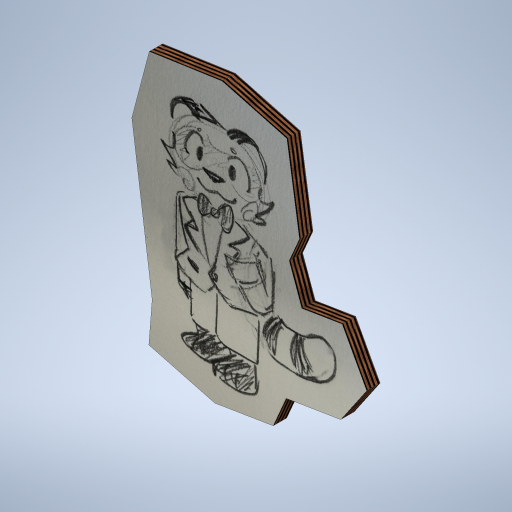
# Autodesk Inventor part: petti
Saved by Autodesk Inventor 2023 (Build 270158000, 158)
## iProperties
Created: 2024-07-02
Part Number: petti
Material: Generic
Document SubType Name: Modeling
Designer: Student-27
Density: 1 g/cm^3
Appearance: Default
Author: Student-27
Autodesk Inventor part; units mm, degrees
ref_plane "YZ Plane" through (0, 0, 0) normal (1, 0, 0) x (0, 1, 0)
ref_plane "XZ Plane" through (0, 0, 0) normal (0, 1, 0) x (-1, 0, 0)
ref_plane "XY Plane" through (0, 0, 0) normal (0, 0, 1) x (1, 0, 0)
sketch "Sketch1" plane through (0, 0, 0) normal (0, 0, 1) x (1, 0, 0)
  line L0 (-7.5953, 9.4076) -> (792.5047, 9.4076) construction
  line L1 (792.5047, 9.4076) -> (792.5047, -1057.3924) construction
  line L2 (792.5047, -1057.3924) -> (-7.5953, -1057.3924) construction
  line L3 (-7.5953, -1057.3924) -> (-7.5953, 9.4076) construction
  line L4 (391.2026, -306.0369) -> (514.2891, -338.9885)
  line L5 (514.2891, -338.9885) -> (538.0727, -491.3852)
  line L6 (538.0727, -491.3852) -> (518.6531, -536.4419)
  line L7 (518.6531, -536.4419) -> (542.5289, -602.5594)
  line L8 (542.5289, -602.5594) -> (618.6657, -590.1287)
  line L9 (618.6657, -590.1287) -> (664.9302, -676.146)
  line L10 (664.9302, -676.146) -> (615.9468, -747.6618)
  line L11 (615.9468, -747.6618) -> (513.1068, -764.4524)
  line L12 (513.1068, -764.4524) -> (488.4994, -821.5458)
  line L13 (488.4994, -821.5458) -> (378.1142, -839.5683)
  line L14 (378.1142, -839.5683) -> (253.8056, -806.7882)
  line L15 (253.8056, -806.7882) -> (260.0674, -729.2793)
  line L16 (260.0674, -729.2793) -> (221.6415, -451.1978)
  line L17 (221.6415, -451.1978) -> (254.5109, -326.5507)
  line L18 (254.5109, -326.5507) -> (391.9348, -306.2329)
  line L19 (221.6415, -306.2329) -> (664.9302, -306.2329)
  line L20 (664.9302, -306.2329) -> (664.9302, -840.0021)
  line L21 (664.9302, -840.0021) -> (221.6415, -840.0021)
  line L22 (221.6415, -840.0021) -> (221.6415, -306.2329)
  point P0 (0, 0)
  dimension "d15" = 533.7692
  dimension "d18" = 443.2887
  constraints: 38 end point, 5 parallel, 2 perpendicular, 2 point on line, 1 horizontal, 2 other
  measures "d15" distance of L21.end L19.start
  measures "d18" distance of L19.start L19.end
extrude "Extrusion1" add sketch "Sketch1" against normal blind 25.4 contours L4 L5 L6 L7 L8 L9 L10 L11 L12 L13 L14 L15 L16 L17 L18
body "Solid1"
